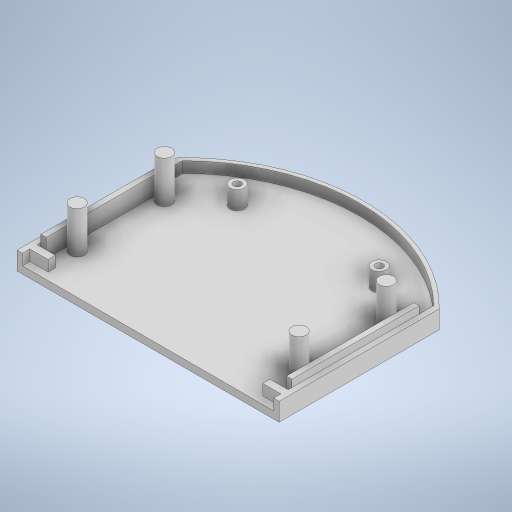
# Autodesk Inventor part: Spiel_Deckel
Saved by Autodesk Inventor 2024 (Build 280153000, 153)
## iProperties
Created: 2024-01-17
Part Number: Spiel_Deckel
Material: Generisch
Document SubType Name: Modeling
Designer: User
Density: 1 g/cm^3
Appearance: Vorgabe
Author: User
Autodesk Inventor part; units mm, degrees
ref_plane "YZ Plane" through (0, 0, 0) normal (1, 0, 0) x (0, 1, 0)
ref_plane "XZ Plane" through (0, 0, 0) normal (0, 1, 0) x (-1, 0, 0)
ref_plane "XY Plane" through (0, 0, 0) normal (0, 0, 1) x (1, 0, 0)
sketch "Skizze1" plane through (0, 0, 0) normal (0, 0, 1) x (1, 0, 0)
  line L0 (-20.1131, -4) -> (51.8869, -4)
  line L1 (51.8869, -4) -> (51.8869, 40)
  line L2 (51.8869, 40) -> (-20.1131, 40)
  line L3 (-20.1131, 40) -> (-20.1131, -4)
  arc A0 (51.8869, 40) -> (-20.1131, 40) centre (15.8869, 5.3013) ccw
  line L4 (50.3869, -4) -> (50.3869, 40)
  line L5 (-18.6131, 40) -> (-18.6131, -4)
  arc A1 (50.3869, 40) -> (-18.6131, 40) centre (15.8869, 5.2581) ccw
  point P0 (0, 0)
  dimension "d0" = 72
  dimension "d1" = 44
  dimension "d2" = 50
  dimension "d3" = 1.5
  dimension "d4" = 1.5
  constraints: 12 end point, 4 point on circle, 4 point on line, 3 parallel, 2 centre point, 1 horizontal, 1 perpendicular
  measures "d0" distance of L2.end L1.end
  measures "d1" distance of L1.end L0.end
  measures "d2" radius of A0
  measures "d3" distance between parallel lines of L1 L4
  measures "d4" distance between parallel lines of L3 L5
extrude "Extrusion1" add sketch "Skizze1" along normal blind 2 contours L5 L2 L4 L0 | A1 L2
extrude "Extrusion2" add sketch "Skizze1" along normal blind 5 contours L3 L2 L5 L0 | A0 L2 A1 | L4 L2 L1 L0
sketch "Skizze2" plane through (0, 0, 2) normal (0, 0, 1) x (1, 0, 0)
  line L0 (50.3869, 40) -> (50.3869, -4) projected
  line L1 (50.3869, -4) -> (43.3869, -4)
  line L2 (-18.6131, 0) -> (-13.6131, 0)
  line L3 (-13.6131, 0) -> (-13.6131, -2)
  line L4 (-13.6131, -2) -> (-18.6131, -2)
  line L5 (-18.6131, -2) -> (-18.6131, 0)
  line L6 (45.3869, 0) -> (50.3869, 0)
  line L7 (50.3869, 0) -> (50.3869, -2)
  line L8 (50.3869, -2) -> (45.3869, -2)
  line L9 (45.3869, -2) -> (45.3869, 0)
  line L10 (-18.6131, -4) -> (50.3869, -4) projected
  circle A0 centre (-14.6131, 7) radius 2
  circle A1 centre (46.3869, 7) radius 2
  circle A2 centre (46.3869, 31) radius 2
  circle A3 centre (-14.6131, 31) radius 2
  line L11 (-18.6131, -4) -> (-18.6131, 40) projected
  circle A4 centre (-3.6131, 40) radius 1.05
  circle A5 centre (-3.6131, 40) radius 2
  circle A6 centre (35.3869, 40) radius 1.05
  circle A7 centre (35.3869, 40) radius 2
  line L12 (50.3869, 1) -> (48.8869, 1)
  line L13 (48.8869, 1) -> (48.8869, 36)
  line L14 (48.8869, 36) -> (50.3869, 36)
  line L15 (50.3869, 36) -> (50.3869, 1)
  line L16 (-18.6131, 36) -> (-17.1131, 36)
  line L17 (-17.1131, 36) -> (-17.1131, 1)
  line L18 (-17.1131, 1) -> (-18.6131, 1)
  line L19 (-18.6131, 1) -> (-18.6131, 36)
  point P0 (0, 0)
  point P1 (45.3869, -1)
  point P2 (-13.6131, -1)
  point P3 (-16.1131, -2)
  point P4 (49.6369, 1)
  point P5 (-17.8631, 1)
  dimension "d40" = 5
  dimension "d41" = 2
  dimension "d43" = 5
  dimension "d44" = 2
  dimension "d45" = 2
  dimension "d46" = 59
  dimension "d52" = 2
  dimension "d53" = 4
  dimension "d54" = 4
  dimension "d55" = 4
  dimension "d56" = 4
  dimension "d57" = 4
  dimension "d58" = 4
  dimension "d59" = 4
  dimension "d60" = 4
  dimension "d61" = 35
  dimension "d62" = 11
  dimension "d63" = 11
  dimension "d64" = 35
  dimension "d69" = 2.1
  dimension "d70" = 4
  dimension "d71" = 2.1
  dimension "d72" = 4
  dimension "d73" = 15
  dimension "d74" = 15
  dimension "d75" = 44
  dimension "d76" = 44
  dimension "d81" = 1.5
  dimension "d82" = 35
  dimension "d83" = 5
  dimension "d84" = 1.5
  dimension "d85" = 35
  dimension "d87" = 5
  constraints: 34 end point, 8 centre point, 8 parallel, 5 horizontal, 5 midpoint, 4 perpendicular, 3 point on line, 2 coincident
  measures "d40" distance of L3.end L4.end
  measures "d41" distance of L2.end L3.end
  measures "d43" distance of L7.end L8.end
  measures "d44" distance between parallel lines of L8 L6
  measures "d45" distance between parallel lines of L1 L8
  measures "d46" distance of point (45.387, -1) point (-13.613, -1)
  measures "d52" distance from line of point (-16.113, -2) L10
  measures "d53" diameter of A0
  measures "d54" diameter of A1
  measures "d55" diameter of A2
  measures "d56" diameter of A3
  measures "d57" distance from line of L11 A3.centre
  measures "d58" distance from line of L11 A0.centre
  measures "d59" distance from line of L0 A1.centre
  measures "d60" distance from line of L0 A2.centre
  measures "d61" distance from line of L10 A2.centre
  measures "d62" distance from line of L10 A1.centre
  measures "d63" distance from line of L10 A0.centre
  measures "d64" distance from line of L10 A3.centre
  measures "d69" diameter of A4
  measures "d70" diameter of A5
  measures "d71" diameter of A6
  measures "d72" diameter of A7
  measures "d73" distance from line of L11 A5.centre
  measures "d74" distance from line of L0 A7.centre
  measures "d75" distance from line of L10 A6.centre
  measures "d76" distance from line of L10 A4.centre
  measures "d81" distance of L13.end L14.end
  measures "d82" distance of L12.end L13.end
  measures "d83" distance from line of L10 point (49.637, 1)
  measures "d84" distance of L17.end L18.end
  measures "d85" distance of L16.end L17.end
  measures "d87" distance from line of L10 point (-17.863, 1)
extrude "Extrusion7" add sketch "Skizze2" along normal blind 3 contours L5 L2 L3 L4 | L0 L8 L9 L6
extrude "Extrusion8" add sketch "Skizze2" along normal blind 11.5 contours A0 | A1 | A2 | A3
extrude "Extrusion9" add sketch "Skizze2" along normal blind 5 contours L11 L16 L17 L18 | L0 L12 L13 L14 | A5 | A7
extrude "Extrusion10" cut sketch "Skizze2" against normal up to next contours A4 | A6
